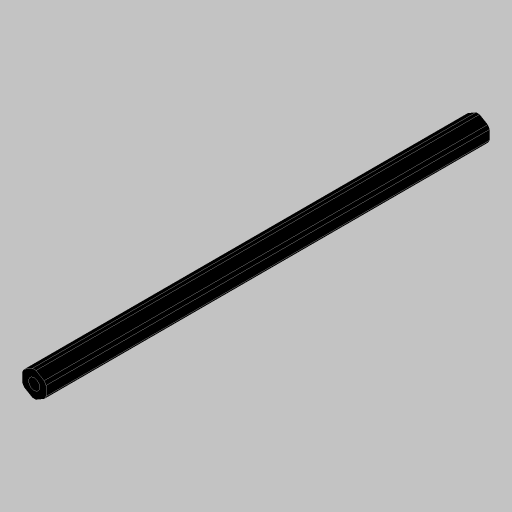
# Autodesk Inventor part: GP5-008
Saved by Autodesk Inventor 2023.5 (Build 275446000, 446)
## iProperties
RuleStatus: InUse
Created: 2025-02-04
Part Number: GP5-008
Material: Aluminum 6061
Document SubType Name: Modeling
Designer: mavericks
Mass: 8.50758 g
Surface Area: 25.7449 cm^2
Volume: 3.15096 cm^3
Density: 2.7 g/cm^3
Appearance: Anodized - Black
AfterDocNew0: SHOW
AfterDocOpen0: SHOW
AfterDocOpen1: size
AfterDocOpen2: thunder
BeforeDocSave0: size
BeforeDocSave1: thunder
AfterFeatureSuppressionChange0: thunder
AfterFeatureSuppressionChange1: size
PartBodyChanged0: thunder
PartBodyChanged1: size
AfterMaterialChange0: thunder
AfterMaterialChange1: size
Author: mavericks
Autodesk Inventor part; units mm, degrees
ref_plane "YZ Plane" through (0, 0, 0) normal (1, 0, 0) x (0, 1, 0)
ref_plane "XZ Plane" through (0, 0, 0) normal (0, 1, 0) x (-1, 0, 0)
ref_plane "XY Plane" through (0, 0, 0) normal (0, 0, 1) x (1, 0, 0)
sketch "Sketch1" plane through (0, 0, 0) normal (0, 0, 1) x (1, 0, 0)
  line L0 (-4.7625, -2.7496) -> (-4.7625, 2.7496)
  line L1 (-4.7625, 2.7496) -> (0, 5.4993)
  line L2 (0, 5.4993) -> (4.7625, 2.7496)
  line L3 (4.7625, 2.7496) -> (4.7625, -2.7496)
  line L4 (4.7625, -2.7496) -> (0, -5.4993)
  line L5 (0, -5.4993) -> (-4.7625, -2.7496)
  point P0 (0, 0)
  point P1 (0, 0)
  dimension "Size" = 9.525
  constraints: 12 end point, 1 coincident, 1 vertical alignment, 13 other
  measures "Size" distance between parallel lines of L3 L0
extrude "Extrusion1" add sketch "Sketch1" along normal mid plane 177.8
sketch "Sketch3" plane through (0, 0, 88.9) normal (0, 0, 1) x (1, 0, 0)
  line L0 (-4.7625, 2.7496) -> (0, 5.4993) construction
  line L1 (0, 5.4993) -> (4.7625, 2.7496) construction
  line L2 (4.7625, 2.7496) -> (4.7625, -2.7496) construction
  line L3 (4.7625, -2.7496) -> (0, -5.4993) construction
  line L4 (0, -5.4993) -> (-4.7625, -2.7496) construction
  line L5 (-4.7625, -2.7496) -> (-4.7625, 2.7496) construction
  point P0 (0, 0)
hole "Hole1" at (0, 0, 88.9) direction (0, 0, -1) diameter 4.4958 end through all
sketch "Sketch4" plane through (0, 0, 88.9) normal (0, 0, 1) x (1, 0, 0)
  circle A0 centre (0, 0) radius 2.2479 construction
  line L0 (-4.7625, 2.7496) -> (0, 5.4993) construction
  line L1 (0, 5.4993) -> (4.7625, 2.7496) construction
  line L2 (4.7625, 2.7496) -> (4.7625, -2.7496) construction
  line L3 (4.7625, -2.7496) -> (0, -5.4993) construction
  line L4 (0, -5.4993) -> (-4.7625, -2.7496) construction
  line L5 (-4.7625, -2.7496) -> (-4.7625, 2.7496) construction
  circle A1 centre (0, 0) radius 5.1245
  circle A2 centre (0, 0) radius 8.89
  dimension "thunder" = 10.2489
  dimension "d16" = 17.78
  constraints: 2 centre point, 2 coincident
  measures "thunder" diameter of A1
  measures "d16" diameter of A2
extrude "Extrusion3" cut sketch "Sketch4" against normal through all
equation "\"bearing\" = 25.4"
body "Solid1"
